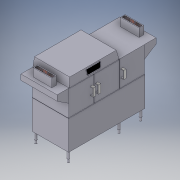
# Autodesk Inventor part: maquinaLAvadoraVajilla480603
Saved by Autodesk Inventor 2018 (Build 220112000, 112)
## iProperties
Created: 2020-04-13
Part Number: maquinaLAvadoraVajilla480603
Material: Generic
Document SubType Name: Modeling
Designer: Jaime
Density: 1 g/cm^3
Appearance: Weld - Stainless Steel
Author: Jaime
Autodesk Inventor part; units mm, degrees
ref_plane "YZ Plane" through (0, 0, 0) normal (1, 0, 0) x (0, 1, 0)
ref_plane "XZ Plane" through (0, 0, 0) normal (0, 1, 0) x (-1, 0, 0)
ref_plane "XY Plane" through (0, 0, 0) normal (0, 0, 1) x (1, 0, 0)
sketch "Sketch1" plane through (0, 0, 0) normal (0, 1, 0) x (-1, 0, 0)
  line L0 (-396.875, 831.85) -> (396.875, 831.85)
  line L1 (396.875, 831.85) -> (396.875, -831.85)
  line L2 (396.875, -831.85) -> (-396.875, -831.85)
  line L3 (-396.875, -831.85) -> (-396.875, 831.85)
  line L4 (-396.875, 831.85) -> (396.875, -831.85) construction
  line L5 (396.875, 831.85) -> (-396.875, -831.85) construction
  point P0 (0, 0)
  dimension "d0" = 793.75
  dimension "d1" = 1663.7
  constraints: 12 end point, 2 midpoint, 2 parallel, 1 horizontal, 1 perpendicular
  measures "d0" distance of L1.end L2.end
  measures "d1" distance of L0.end L1.end
extrude "Extrusion1" add sketch "Sketch1" along normal mid plane 638.175
sketch "Supports" plane through (0, -319.0875, 0) normal (0, -1, 0) x (1, 0, 0)
  line L0 (396.875, 831.85) -> (-396.875, 831.85) construction
  line L1 (-396.875, 831.85) -> (-396.875, -831.85) construction
  line L2 (-396.875, -831.85) -> (396.875, -831.85) construction
  line L3 (396.875, -831.85) -> (396.875, 831.85) construction
  point P0 (0, 0)
sketch "Sketch3" plane through (0, 319.0875, 0) normal (0, 1, 0) x (1, 0, 0)
  line L0 (-396.875, -831.85) -> (396.875, -831.85) construction
  line L1 (396.875, -831.85) -> (396.875, 831.85) construction
  line L2 (396.875, 831.85) -> (-396.875, 831.85) construction
  line L3 (-396.875, 831.85) -> (-396.875, -831.85) construction
  line L4 (-396.875, -825.5) -> (396.875, -825.5)
  line L5 (396.875, -825.5) -> (396.875, 825.5)
  line L6 (396.875, 825.5) -> (-396.875, 825.5)
  line L7 (-396.875, 825.5) -> (-396.875, -825.5)
  line L8 (-396.875, -825.5) -> (396.875, 825.5) construction
  line L9 (396.875, -825.5) -> (-396.875, 825.5) construction
  point P0 (0, 0)
  dimension "d4" = 793.75
  dimension "d5" = 1651
  constraints: 12 end point, 2 midpoint, 2 parallel, 1 horizontal, 1 perpendicular
  measures "d4" distance of L6.end L5.end
  measures "d5" distance of L5.end L4.end
extrude "Extrusion2" add sketch "Sketch3" along normal blind 571.5
sketch "Sketch4" plane through (396.875, -319.0875, -831.85) normal (1, 0, 0) x (0, 0, -1)
  line L0 (0, 638.175) -> (0, 0) construction
  line L1 (-6.35, 638.175) -> (0, 638.175) construction
  line L2 (-6.35, 638.175) -> (-6.35, 1209.675) construction
  line L3 (-1657.35, 1209.675) -> (-6.35, 1209.675) construction
  line L4 (-1657.35, 638.175) -> (-1657.35, 1209.675) construction
  line L5 (-1663.7, 638.175) -> (-1657.35, 638.175) construction
  line L6 (-1663.7, 0) -> (-1663.7, 638.175) construction
  line L7 (0, 0) -> (-1663.7, 0) construction
  line L8 (-1657.35, 638.175) -> (-1657.35, 1209.675) construction
  line L9 (-1657.35, 1209.675) -> (-6.35, 1209.675) construction
  line L10 (-6.35, 1209.675) -> (-6.35, 638.175) construction
  line L11 (-1657.35, 638.175) -> (-1657.35, 1209.675) construction
  line L12 (-1657.35, 1209.675) -> (-6.35, 1209.675) construction
  line L13 (-1657.35, 1209.675) -> (-1107.0167, 1209.675) construction
  line L14 (-1657.35, 1209.675) -> (-1107.0167, 1209.675) construction
  line L15 (-1107.0167, 1209.675) -> (-556.6833, 1209.675) construction
  line L16 (-1107.0167, 1209.675) -> (-556.6833, 1209.675) construction
  line L17 (-556.6833, 1209.675) -> (-6.35, 1209.675) construction
  line L18 (-1107.0167, 1209.675) -> (-1107.0167, 638.175) construction
  line L19 (-556.6833, 1209.675) -> (-556.6833, 638.175) construction
  line L20 (-1113.3667, 638.175) -> (-1100.6667, 638.175)
  line L21 (-1100.6667, 650.875) -> (-1100.6667, 1209.675)
  line L22 (-1100.6667, 1209.675) -> (-1113.3667, 1209.675)
  line L23 (-1113.3667, 1209.675) -> (-1113.3667, 650.875)
  line L24 (-1113.3667, 638.175) -> (-1100.6667, 1209.675) construction
  line L25 (-1100.6667, 638.175) -> (-1113.3667, 1209.675) construction
  line L26 (-563.0333, 638.175) -> (-550.3333, 638.175)
  line L27 (-550.3333, 650.875) -> (-550.3333, 1209.675)
  line L28 (-550.3333, 1209.675) -> (-563.0333, 1209.675)
  line L29 (-563.0333, 1209.675) -> (-563.0333, 650.875)
  line L30 (-563.0333, 638.175) -> (-550.3333, 1209.675) construction
  line L31 (-550.3333, 638.175) -> (-563.0333, 1209.675) construction
  line L32 (-6.35, 638.175) -> (-6.35, 650.875) construction
  line L33 (-6.35, 638.175) -> (6.35, 638.175) construction
  line L34 (-1657.35, 638.175) -> (-6.35, 638.175)
  line L35 (-6.35, 638.175) -> (-6.35, 650.875)
  line L36 (-1657.35, 650.875) -> (-1657.35, 638.175)
  line L37 (-1113.0844, 650.875) -> (-1657.35, 650.875)
  line L38 (-6.35, 638.175) -> (-1107.0167, 638.175) construction
  line L39 (-1113.3667, 638.175) -> (-1657.35, 638.175) construction
  line L40 (-6.35, 650.875) -> (-550.6156, 650.875)
  line L41 (-562.7511, 650.875) -> (-1100.9489, 650.875)
  point P0 (-831.85, 319.0875)
  point P1 (-1107.0167, 923.925)
  point P2 (-556.6833, 923.925)
  dimension "d8" = 550.3333
  dimension "d9" = 0
  dimension "d10" = 550.3333
  dimension "d11" = 0
  dimension "d12" = 12.7
  dimension "d13" = 12.7
  dimension "d16" = 12.7
  dimension "d17" = 90
  dimension "d18" = 1.273
  dimension "d19" = 638.175
  dimension "d20" = 650.875
  dimension "d21" = 638.175
  dimension "d22" = 650.875
  constraints: 64 end point, 12 parallel, 10 point on line, 8 horizontal, 8 perpendicular, 7 midpoint, 3 equal length, 2 collinear, 1 vertical
  measures "d8" distance of L3.start L13.end
  measures "d9" distance between parallel lines of L13 L14
  measures "d10" distance of L14.end L15.end
  measures "d11" distance between parallel lines of L15 L16
  measures "d12" distance of L22.end L21.end
  measures "d13" distance of L28.end L27.end
  measures "d16" distance of L1.start L32.end
  measures "d17" angle of L33 L32
  measures "d18" angle of L0 L30
  measures "d19" distance between parallel lines of L7 L26
  measures "d20" distance between parallel lines of L7 L41
  measures "d21" distance between parallel lines of L7 L34
  measures "d22" distance between parallel lines of L7 L37
extrude "Extrusion3" cut sketch "Sketch4" against normal blind 12.7
sketch "Sketch5" plane through (-396.875, -319.0875, 831.85) normal (-1, 0, 0) x (0, 0, 1)
  line L0 (0, 638.175) -> (0, 0) construction
  line L1 (-6.35, 638.175) -> (0, 638.175) construction
  line L2 (-6.35, 638.175) -> (-6.35, 1209.675) construction
  line L3 (-1657.35, 1209.675) -> (-6.35, 1209.675) construction
  line L4 (-1657.35, 638.175) -> (-1657.35, 1209.675) construction
  line L5 (-1663.7, 638.175) -> (-1657.35, 638.175) construction
  line L6 (-1663.7, 638.175) -> (-1663.7, 0) construction
  line L7 (0, 0) -> (-1663.7, 0) construction
  line L8 (-1657.35, 638.175) -> (-6.35, 638.175) construction
  line L9 (-1657.35, 638.175) -> (-1657.35, 1209.675) projected
  line L10 (-1657.35, 1209.675) -> (-1657.35, 923.925)
  line L11 (-1657.35, 1209.675) -> (-1371.6, 1209.675) construction
  line L12 (-1657.35, 1209.675) -> (-1911.35, 1209.675)
  line L13 (-1657.35, 1209.675) -> (-1403.35, 1209.675) construction
  line L14 (-1911.35, 1209.675) -> (-1911.35, 1089.025)
  line L15 (-1911.35, 1089.025) -> (-1657.35, 923.925)
  line L16 (-1657.35, 1209.675) -> (-6.35, 1209.675) construction
  line L17 (-1657.35, 1209.675) -> (-831.85, 1209.675) construction
  line L18 (-1657.35, 1209.675) -> (-831.85, 1209.675) construction
  line L19 (-831.85, 1209.675) -> (-831.85, 638.175) construction
  line L20 (-6.35, 1209.675) -> (-6.35, 923.925)
  line L21 (-6.35, 1209.675) -> (247.65, 1209.675)
  line L22 (247.65, 1209.675) -> (247.65, 1089.025)
  line L23 (247.65, 1089.025) -> (-6.35, 923.925)
  point P0 (-831.85, 319.0875)
  dimension "d23" = 285.75
  dimension "d24" = 90
  dimension "d25" = 254
  dimension "d26" = 180
  dimension "d27" = 120.65
  dimension "d28" = 90
  dimension "d30" = 825.5
  dimension "d31" = 0
  constraints: 26 end point, 4 horizontal, 3 equal length, 3 symmetric about line, 2 perpendicular, 1 collinear, 1 midpoint
  measures "d23" distance of L3.start L10.end
  measures "d24" angle of L10 L11
  measures "d25" distance of L3.start L12.end
  measures "d26" angle of L12 L13
  measures "d27" distance of L12.end L14.end
  measures "d28" angle of L14 L12
  measures "d30" distance of L3.start L17.end
  measures "d31" distance between parallel lines of L17 L18
extrude "Extrusion4" add sketch "Sketch5" against normal blind 790.575
sketch "Sketch7" plane through (0, 890.5875, 0) normal (0, 1, 0) x (1, 0, 0)
  line L0 (396.875, 268.8167) -> (384.175, 268.8167) construction
  line L1 (384.175, 268.8167) -> (384.175, 281.5167) construction
  line L2 (384.175, 281.5167) -> (396.875, 281.5167) construction
  line L3 (396.875, 281.5167) -> (396.875, 825.5) construction
  line L4 (396.875, 825.5) -> (393.7, 825.5) construction
  line L5 (393.7, 1079.5) -> (393.7, 825.5) construction
  line L6 (-396.875, 1079.5) -> (393.7, 1079.5) construction
  line L7 (-396.875, 1079.5) -> (-396.875, -1079.5) construction
  line L8 (-396.875, -1079.5) -> (393.7, -1079.5) construction
  line L9 (393.7, -825.5) -> (393.7, -1079.5) construction
  line L10 (393.7, -825.5) -> (396.875, -825.5) construction
  line L11 (396.875, -825.5) -> (396.875, -281.5167) construction
  line L12 (396.875, -281.5167) -> (384.175, -281.5167) construction
  line L13 (384.175, -281.5167) -> (384.175, -268.8167) construction
  line L14 (384.175, -268.8167) -> (396.875, -268.8167) construction
  line L15 (396.875, -268.8167) -> (396.875, 268.8167) construction
  line L16 (-396.875, 825.5) -> (393.7, 825.5) construction
  line L17 (393.7, -825.5) -> (-396.875, -825.5) construction
  line L18 (-396.875, 1079.5) -> (393.7, 1079.5) construction
  line L19 (-1.5875, 1079.5) -> (-1.5875, 825.5) construction
  line L20 (-396.875, 825.5) -> (384.175, 825.5) construction
  line L21 (393.7, -825.5) -> (396.875, -825.5) construction
  line L22 (-396.875, -825.5) -> (393.7, -825.5) construction
  line L23 (393.7, 825.5) -> (-396.875, 825.5) construction
  line L24 (-396.875, -831.85) -> (-396.875, 831.85) projected
  line L25 (-396.875, -825.5) -> (-396.875, -831.85) projected
  line L26 (-396.875, -825.5) -> (393.7, -1079.5) construction
  line L27 (393.7, -825.5) -> (-396.875, -1079.5) construction
  line L28 (0, 0) -> (762, 0) construction
  line L29 (0, 0) -> (762, 0) construction
  line L30 (-396.875, -1079.5) -> (-396.875, 1079.5) construction
  line L31 (-396.875, 1079.5) -> (393.7, 1079.5) construction
  line L32 (393.7, 825.5) -> (393.7, 1079.5) construction
  line L33 (393.7, 825.5) -> (396.875, 825.5) construction
  line L34 (396.875, 825.5) -> (396.875, 281.5167) construction
  line L35 (393.7, 825.5) -> (-396.875, 825.5) construction
  line L36 (393.7, 825.5) -> (396.875, 825.5) construction
  line L37 (-396.875, 825.5) -> (393.7, 825.5) construction
  line L38 (-396.875, 831.85) -> (-396.875, -831.85)
  line L39 (-396.875, 825.5) -> (-396.875, 831.85)
  line L40 (-396.875, 825.5) -> (393.7, 1079.5) construction
  line L41 (393.7, 825.5) -> (-396.875, 1079.5) construction
  line L42 (-204.7875, 901.7) -> (201.6125, 901.7)
  line L43 (201.6125, 901.7) -> (201.6125, 1003.3)
  line L44 (201.6125, 1003.3) -> (-204.7875, 1003.3)
  line L45 (-204.7875, 1003.3) -> (-204.7875, 901.7)
  line L46 (-204.7875, 901.7) -> (201.6125, 1003.3) construction
  line L47 (201.6125, 901.7) -> (-204.7875, 1003.3) construction
  line L48 (-204.7875, -1003.3) -> (201.6125, -1003.3)
  line L49 (201.6125, -1003.3) -> (201.6125, -901.7)
  line L50 (201.6125, -901.7) -> (-204.7875, -901.7)
  line L51 (-204.7875, -901.7) -> (-204.7875, -1003.3)
  line L52 (-204.7875, -1003.3) -> (201.6125, -901.7) construction
  line L53 (201.6125, -1003.3) -> (-204.7875, -901.7) construction
  point P0 (-1.5875, 952.5)
  point P1 (-1.5875, -952.5)
  dimension "d34" = 762
  dimension "d35" = 0
  dimension "d36" = 406.4
  dimension "d37" = 101.6
  dimension "d38" = 406.4
  dimension "d39" = 101.6
  constraints: 62 end point, 7 midpoint, 5 perpendicular, 4 horizontal, 4 parallel, 4 symmetric about line, 1 collinear, 1 point on line
  measures "d34" distance of L28.start L28.end
  measures "d35" distance between parallel lines of L28 L29
  measures "d36" distance of L44.end L43.end
  measures "d37" distance of L43.end L42.end
  measures "d38" distance of L50.end L49.end
  measures "d39" distance of L49.end L48.end
extrude "Extrusion5" add sketch "Sketch7" along normal blind 177.8
sketch "Sketch8" plane through (396.875, 331.7875, -268.8167) normal (1, 0, 0) x (0, 0, -1)
  line L0 (-550.3333, 0) -> (-550.3333, 558.8) construction
  line L1 (-1094.3167, 558.8) -> (-550.3333, 558.8) construction
  line L2 (-1094.3167, 0) -> (-1094.3167, 558.8) construction
  line L3 (-1094.3167, 0) -> (-550.3333, 0) construction
  line L4 (0, 0) -> (0, 558.8) construction
  line L5 (-537.6333, 558.8) -> (0, 558.8) construction
  line L6 (-537.6333, 558.8) -> (-537.6333, 0) construction
  line L7 (-537.6333, 0) -> (0, 0) construction
  line L8 (556.6833, -12.7) -> (-1094.3167, -12.7) construction
  line L9 (556.6833, 0) -> (556.6833, -12.7) projected
  line L10 (12.7, 0) -> (556.6833, 0) construction
  line L11 (12.7, 558.8) -> (12.7, 0) construction
  line L12 (0, 558.8) -> (12.7, 558.8) construction
  line L13 (0, 0) -> (0, 558.8) construction
  line L14 (-537.6333, 0) -> (0, 0) construction
  line L15 (-537.6333, 558.8) -> (-537.6333, 0) construction
  line L16 (-550.3333, 558.8) -> (-537.6333, 558.8) construction
  line L17 (-550.3333, 0) -> (-550.3333, 558.8) construction
  line L18 (-1094.3167, 0) -> (-550.3333, 0) construction
  line L19 (-1094.3167, -12.7) -> (-1094.3167, 0) construction
  line L20 (-543.9833, 558.8) -> (-543.9833, 736.6) construction
  line L21 (-543.9833, 558.8) -> (-366.1833, 558.8) construction
  line L22 (-543.9833, 736.6) -> (-35.9833, 736.6)
  line L23 (-543.9833, 736.6) -> (-35.9833, 736.6) construction
  line L24 (0, 0) -> (0, 558.8) construction
  line L25 (-35.9833, 736.6) -> (0, 558.8)
  line L26 (0, 558.8) -> (-543.9833, 558.8)
  line L27 (-550.3333, 558.8) -> (-537.6333, 558.8) projected
  line L28 (-543.9833, 736.6) -> (-543.9833, 558.8) construction
  line L29 (-537.6333, 0) -> (-537.6333, 558.8) construction
  line L30 (6.35, 558.8) -> (-537.6333, 558.8) construction
  line L31 (-1087.9667, 0) -> (-1087.9667, 558.8) construction
  line L32 (-550.3333, 558.8) -> (-1087.9667, 558.8) construction
  line L33 (-550.3333, 558.8) -> (-550.3333, 0) construction
  line L34 (-1100.6667, 558.8) -> (-1100.6667, 0) construction
  line L35 (-1087.9667, 558.8) -> (-1100.6667, 558.8) construction
  line L36 (-1087.9667, 0) -> (-1087.9667, 558.8) construction
  line L37 (-550.3333, 558.8) -> (-550.3333, 0) construction
  line L38 (-537.6333, 558.8) -> (-550.3333, 558.8) construction
  line L39 (-537.6333, 0) -> (-537.6333, 558.8) construction
  line L40 (-543.9833, 558.8) -> (-721.7833, 558.8) construction
  line L41 (-543.9833, 736.6) -> (-1051.9833, 736.6)
  line L42 (-543.9833, 736.6) -> (-1051.9833, 736.6) construction
  line L43 (-1087.9667, 0) -> (-1087.9667, 558.8)
  line L44 (-1051.9833, 736.6) -> (-1087.9667, 558.8)
  line L45 (-1087.9667, 558.8) -> (-543.9833, 558.8)
  line L46 (-537.6333, 558.8) -> (-550.3333, 558.8)
  point P0 (-268.8167, -331.7875)
  dimension "d42" = 177.8
  dimension "d43" = 90
  dimension "d44" = 508
  dimension "d45" = 0
  constraints: 50 end point, 18 symmetric about line, 3 horizontal, 2 collinear, 2 equal length, 1 midpoint, 1 vertical
  measures "d42" distance of L20.start L20.end
  measures "d43" angle of L21 L20
  measures "d44" distance of L20.end L22.end
  measures "d45" distance between parallel lines of L22 L23
extrude "Extrusion6" add sketch "Sketch8" against normal blind 793.75
sketch "Sketch9" plane through (396.875, 331.7875, 825.5) normal (1, 0, 0) x (0, 0, -1)
  line L0 (1094.3167, 0) -> (1094.3167, 558.8) construction
  line L1 (1094.3167, 558.8) -> (1058.3333, 736.6) construction
  line L2 (1058.3333, 736.6) -> (42.3333, 736.6) construction
  line L3 (42.3333, 736.6) -> (6.35, 558.8) construction
  line L4 (0, 558.8) -> (6.35, 558.8) construction
  line L5 (0, 0) -> (0, 558.8) construction
  line L6 (0, 0) -> (543.9833, 0) construction
  line L7 (543.9833, 0) -> (543.9833, 558.8) construction
  line L8 (543.9833, 558.8) -> (556.6833, 558.8) construction
  line L9 (556.6833, 558.8) -> (556.6833, 0) construction
  line L10 (556.6833, 0) -> (1094.3167, 0) construction
  line L11 (0, 558.8) -> (1104.9, 558.8)
  line L12 (1104.9, 558.8) -> (1104.9, 546.1)
  line L13 (1104.9, 546.1) -> (0, 546.1)
  line L14 (0, 546.1) -> (0, 558.8)
  point P0 (825.5, -331.7875)
  dimension "d48" = 1104.9
  dimension "d49" = 12.7
  constraints: 8 end point, 2 parallel, 1 horizontal, 1 perpendicular
  measures "d48" distance of L12.end L13.end
  measures "d49" distance of L11.end L12.end
extrude "Extrusion7" cut sketch "Sketch9" against normal blind 12.7
sketch "Sketch10" plane through (396.875, 1068.3875, 783.1667) normal (1, 0, 0) x (0, 0, -1)
  line L0 (-35.9833, -177.8) -> (1051.9833, -177.8) construction
  line L1 (1051.9833, -177.8) -> (1016, 0) construction
  line L2 (1016, 0) -> (0, 0) construction
  line L3 (0, 0) -> (-35.9833, -177.8) construction
  line L4 (1016, 0) -> (0, 0) projected
  line L5 (0, 0) -> (1051.9833, -177.8) construction
  line L6 (-35.9833, -177.8) -> (-296.3333, -177.8) projected
  line L7 (-35.9833, -177.8) -> (1016, 0) construction
  line L8 (384.1714, -136.6592) -> (631.8286, -136.6592)
  line L9 (660.4, -136.6592) -> (660.4, -35.0592) construction
  line L10 (645.2647, -35.0592) -> (370.7353, -35.0592)
  line L11 (355.6, -35.0592) -> (355.6, -136.6592) construction
  line L12 (355.6, -136.6592) -> (660.4, -35.0592) construction
  line L13 (660.4, -136.6592) -> (355.6, -35.0592) construction
  line L14 (358.2282, -49.9645) -> (371.6643, -126.1645)
  line L15 (355.6, -35.0592) -> (482.6, -35.0592) construction
  line L16 (508, -85.8592) -> (508, -35.0592) construction
  line L17 (657.7718, -49.9645) -> (644.3357, -126.1645)
  arc A0 (370.7353, -35.0592) -> (358.2282, -49.9645) centre (370.7353, -47.7592) ccw
  arc A1 (657.7718, -49.9645) -> (645.2647, -35.0592) centre (645.2647, -47.7592) ccw
  arc A2 (371.6643, -126.1645) -> (384.1714, -136.6592) centre (384.1714, -123.9592) ccw
  arc A3 (631.8286, -136.6592) -> (644.3357, -126.1645) centre (631.8286, -123.9592) ccw
  line L18 (370.7353, -22.3592) -> (645.2647, -22.3592)
  arc A4 (670.2788, -52.1698) -> (645.2647, -22.3592) centre (645.2647, -47.7592) ccw
  line L19 (670.2788, -52.1698) -> (656.8427, -128.3698)
  arc A5 (631.8286, -149.3592) -> (656.8427, -128.3698) centre (631.8286, -123.9592) ccw
  line L20 (631.8286, -149.3592) -> (384.1714, -149.3592)
  arc A6 (359.1573, -128.3698) -> (384.1714, -149.3592) centre (384.1714, -123.9592) ccw
  line L21 (359.1573, -128.3698) -> (345.7212, -52.1698)
  arc A7 (370.7353, -22.3592) -> (345.7212, -52.1698) centre (370.7353, -47.7592) ccw
  point P0 (783.1667, -1068.3875)
  point P1 (373.5148, -136.6592)
  point P2 (642.4852, -136.6592)
  dimension "d56" = 304.8
  dimension "d57" = 101.6
  dimension "d59" = 80
  dimension "d60" = 12.7
  dimension "d61" = 12.7
  dimension "d62" = 12.7
  constraints: 32 end point, 16 point on circle, 11 point on line, 8 centre point, 8 tangent, 3 midpoint, 3 parallel, 2 equal radius, 2 horizontal, 1 perpendicular, 1 symmetric about line, 7 other
  measures "d56" distance of L11.start L9.end
  measures "d57" distance of L9.end L9.start
  measures "d59" angle of L14 L15
  measures "d60" radius of A0
  measures "d61" radius of A1
  measures "d62" distance between parallel lines of L10 L18
ref_plane "Work Plane1" through (371.475, 1068.3875, 783.1667) normal (1, 0, 0) x (0, 0, -1)
sketch "Sketch11" plane through (-396.875, 319.0875, 825.5) normal (0, 0, 1) x (1, 0, 0)
  line L0 (793.75, 749.3) -> (793.75, 571.5) construction
  line L1 (793.75, 749.3) -> (0, 749.3) construction
  line L2 (0, 571.5) -> (0, 749.3) construction
  line L3 (781.05, 571.5) -> (0, 571.5) construction
  line L4 (793.75, 571.5) -> (781.05, 571.5) construction
  line L5 (793.75, 571.5) -> (781.05, 571.5) projected
  line L6 (793.75, 571.5) -> (768.2033, 749.3)
  line L7 (793.75, 749.3) -> (0, 749.3) projected
  line L8 (793.75, 749.3) -> (768.2033, 749.3)
  line L9 (793.75, 571.5) -> (793.75, 749.3) projected
  line L10 (793.75, 749.3) -> (793.75, 571.5)
  point P0 (396.875, -319.0875)
  dimension "d53" = 98.176
  constraints: 6 end point, 1 collinear, 1 point on line, 1 vertical
  measures "d53" angle of L7 L6
extrude "Extrusion8" cut sketch "Sketch11" against normal blind 1092.2
extrude "Extrusion9" cut sketch "Sketch10" against normal blind 76.2
sketch "Sketch12" plane through (0, 1068.3875, 0) normal (0, 1, 0) x (1, 0, 0)
  line L0 (-204.7875, 901.7) -> (201.6125, 901.7) construction
  line L1 (-204.7875, 901.7) -> (201.6125, 901.7) construction
  line L2 (201.6125, 901.7) -> (201.6125, 1003.3) construction
  line L3 (201.6125, 1003.3) -> (-204.7875, 1003.3) construction
  line L4 (-204.7875, 1003.3) -> (-204.7875, 901.7) construction
  line L5 (-204.7875, -1003.3) -> (201.6125, -1003.3) construction
  line L6 (201.6125, -1003.3) -> (201.6125, -901.7) construction
  line L7 (201.6125, -901.7) -> (-204.7875, -901.7) construction
  line L8 (-204.7875, -901.7) -> (-204.7875, -1003.3) construction
  line L9 (-204.7875, -1003.3) -> (201.6125, -901.7) construction
  line L10 (-204.7875, -1003.3) -> (201.6125, -1003.3) construction
  line L11 (201.6125, -1003.3) -> (-204.7875, -901.7) construction
  line L12 (188.9125, -985.52) -> (-192.0875, -985.52)
  line L13 (-192.0875, -985.52) -> (-192.0875, -919.48)
  line L14 (-192.0875, -919.48) -> (188.9125, -919.48)
  line L15 (188.9125, -919.48) -> (188.9125, -985.52)
  line L16 (188.9125, -985.52) -> (-192.0875, -919.48) construction
  line L17 (-192.0875, -985.52) -> (188.9125, -919.48) construction
  line L18 (-204.7875, 901.7) -> (-204.7875, 1003.3) construction
  line L19 (201.6125, 1003.3) -> (-204.7875, 901.7) construction
  line L20 (201.6125, 1003.3) -> (-204.7875, 1003.3) construction
  line L21 (-204.7875, 1003.3) -> (201.6125, 901.7) construction
  line L22 (188.9125, 919.48) -> (-192.0875, 919.48)
  line L23 (-192.0875, 919.48) -> (-192.0875, 985.52)
  line L24 (-192.0875, 985.52) -> (188.9125, 985.52)
  line L25 (188.9125, 985.52) -> (188.9125, 919.48)
  line L26 (188.9125, 919.48) -> (-192.0875, 985.52) construction
  line L27 (-192.0875, 919.48) -> (188.9125, 985.52) construction
  point P0 (0, 0)
  point P1 (-1.5875, -952.5)
  point P2 (-1.5875, 952.5)
  dimension "d65" = 381
  dimension "d66" = 66.04
  dimension "d67" = 381
  dimension "d68" = 66.04
  constraints: 32 end point, 6 midpoint, 4 parallel, 2 horizontal, 2 perpendicular
  measures "d65" distance of L13.end L14.end
  measures "d66" distance of L12.end L13.end
  measures "d67" distance of L23.end L24.end
  measures "d68" distance of L22.end L23.end
extrude "Extrusion10" cut sketch "Sketch12" against normal blind 76.2
sketch "Sketch13" plane through (0, -319.0875, 0) normal (0, -1, 0) x (1, 0, 0)
  line L0 (396.875, 831.85) -> (-396.875, 831.85) construction
  line L1 (-396.875, 831.85) -> (-396.875, -831.85) construction
  line L2 (-396.875, -831.85) -> (396.875, -831.85) construction
  line L3 (396.875, -831.85) -> (396.875, 831.85) construction
  line L4 (396.875, 281.5167) -> (396.875, 825.5) construction
  line L5 (396.875, 825.5) -> (396.875, 281.5167) construction
  line L6 (396.875, -268.8167) -> (396.875, 268.8167) construction
  line L7 (396.875, 268.8167) -> (396.875, -268.8167) construction
  line L8 (396.875, 825.5) -> (396.875, 281.5167) construction
  line L9 (396.875, 825.5) -> (396.875, 281.5167) construction
  line L10 (384.175, 825.5) -> (396.875, 825.5) construction
  line L11 (384.175, 825.5) -> (384.175, 281.5167) construction
  line L12 (396.875, 281.5167) -> (384.175, 281.5167) construction
  line L13 (396.875, 268.8167) -> (396.875, -268.8167) construction
  line L14 (396.875, 268.8167) -> (384.175, 268.8167) construction
  line L15 (384.175, 268.8167) -> (384.175, -268.8167) construction
  line L16 (396.875, -268.8167) -> (384.175, -268.8167) construction
  line L17 (-396.875, -268.8167) -> (384.175, -268.8167) construction
  line L18 (396.875, -268.8167) -> (-396.875, -268.8167) construction
  line L19 (384.175, -268.8167) -> (384.175, 268.8167) construction
  line L20 (384.175, -268.8167) -> (-396.875, -831.85) construction
  line L21 (-396.875, -1079.5) -> (-396.875, -268.8167) construction
  line L22 (396.875, -831.85) -> (396.875, 831.85) construction
  line L23 (-396.875, -268.8167) -> (396.875, -831.85) construction
  line L24 (-358.8006, -313.113) -> (352.3994, -313.113) construction
  line L25 (352.3994, -313.113) -> (352.3994, -783.013) construction
  line L26 (352.3994, -783.013) -> (-358.8006, -783.013) construction
  line L27 (-358.8006, -783.013) -> (-358.8006, -313.113) construction
  line L28 (-358.8006, -313.113) -> (352.3994, -783.013) construction
  line L29 (352.3994, -313.113) -> (-358.8006, -783.013) construction
  circle A0 centre (352.3994, -313.113) radius 25.4
  circle A1 centre (352.3994, -783.013) radius 25.4
  circle A2 centre (-358.8006, -313.113) radius 25.4
  circle A3 centre (-358.8006, -783.013) radius 25.4
  line L30 (352.3994, -783.013) -> (352.3994, 791.787) construction
  line L31 (352.3994, -783.013) -> (1927.1994, -783.013) construction
  line L32 (-358.8006, -783.013) -> (-358.8006, 791.787) construction
  line L33 (-358.8006, -783.013) -> (1215.9994, -783.013) construction
  circle A4 centre (352.3994, 791.787) radius 25.4
  circle A5 centre (-358.8006, 791.787) radius 25.4
  point P0 (0, 0)
  point P1 (-3.2006, -548.063)
  dimension "d71" = 711.2
  dimension "d72" = 469.9
  dimension "d73" = 50.8
  dimension "d74" = 50.8
  dimension "d75" = 50.8
  dimension "d76" = 50.8
  dimension "d77" = 1574.8
  dimension "d78" = 90
  dimension "d79" = 1574.8
  dimension "d80" = 90
  dimension "d81" = 50.8
  dimension "d82" = 50.8
  constraints: 26 end point, 6 centre point, 6 coincident, 3 horizontal, 3 perpendicular, 2 midpoint, 2 parallel, 2 point on line, 2 vertical, 1 collinear, 1 other
  measures "d71" distance of L25.end L26.end
  measures "d72" distance of L24.end L25.end
  measures "d73" diameter of A0
  measures "d74" diameter of A1
  measures "d75" diameter of A2
  measures "d76" diameter of A3
  measures "d77" distance of L30.start L30.end
  measures "d78" angle of L31 L30
  measures "d79" distance of L32.start L32.end
  measures "d80" angle of L33 L32
  measures "d81" diameter of A4
  measures "d82" diameter of A5
extrude "Extrusion11" add sketch "Sketch13" along normal blind 152.4
sketch "Sketch14" plane through (352.3994, -471.4875, -313.113) normal (0, -1, 0) x (1, 0, 0)
  line L0 (18.9289, 1096.2797) -> (-749.2744, 1096.2797) construction
  circle A0 centre (0, 1104.9) radius 25.4 construction
  circle A1 centre (0, 1104.9) radius 25.4 construction
  circle A2 centre (-711.2, 0) radius 25.4 construction
  circle A3 centre (0, 0) radius 25.4 construction
  circle A4 centre (0, -469.9) radius 25.4 construction
  circle A5 centre (-711.2, -469.9) radius 25.4 construction
  circle A6 centre (-711.2, 1104.9) radius 25.4 construction
  line L1 (44.4756, 1144.963) -> (-749.2744, 1144.963) construction
  line L2 (-749.2744, 1144.963) -> (-749.2744, -518.737) construction
  line L3 (-749.2744, -518.737) -> (44.4756, -518.737) construction
  line L4 (44.4756, -518.737) -> (44.4756, 1144.963) construction
  circle A7 centre (0, -469.9) radius 20.32
  circle A8 centre (0, 0) radius 20.32
  circle A9 centre (-711.2, -469.9) radius 20.32
  circle A10 centre (-711.2, 0) radius 20.32
  circle A11 centre (-711.2, 1104.9) radius 20.32
  circle A12 centre (0, 1104.9) radius 20.32
  point P0 (-352.3994, 313.113)
  dimension "d85" = 40.64
  dimension "d86" = 40.64
  dimension "d87" = 40.64
  dimension "d88" = 40.64
  dimension "d89" = 40.64
  dimension "d90" = 40.64
  constraints: 6 centre point, 6 coincident
  measures "d85" diameter of A7
  measures "d86" diameter of A8
  measures "d87" diameter of A9
  measures "d88" diameter of A10
  measures "d89" diameter of A11
  measures "d90" diameter of A12
extrude "Extrusion12" add sketch "Sketch14" along normal blind 73.025
sketch "Sketch15" plane through (396.875, 331.7875, 825.5) normal (1, 0, 0) x (0, 0, -1)
  line L0 (543.9833, 546.1) -> (0, 546.1) construction
  line L1 (0, 0) -> (0, 546.1) construction
  line L2 (0, 0) -> (543.9833, 0) construction
  line L3 (543.9833, 0) -> (543.9833, 546.1) construction
  line L4 (1094.3167, 546.1) -> (556.6833, 546.1) construction
  line L5 (556.6833, 546.1) -> (556.6833, 0) construction
  line L6 (556.6833, 0) -> (1094.3167, 0) construction
  line L7 (1094.3167, 0) -> (1094.3167, 546.1) construction
  line L8 (1107.0167, 558.8) -> (1107.0167, 0) construction
  line L9 (1107.0167, 0) -> (1651, 0) construction
  line L10 (1651, 0) -> (1651, 558.8) construction
  line L11 (1107.0167, 558.8) -> (1651, 558.8) construction
  line L12 (543.9833, 546.1) -> (543.9833, 273.05) construction
  line L13 (543.9833, 0) -> (543.9833, 546.1) construction
  line L14 (543.9833, 273.05) -> (556.6833, 273.05) construction
  line L15 (556.6833, 546.1) -> (556.6833, 0) construction
  line L16 (1107.0167, 558.8) -> (1107.0167, 0) construction
  line L17 (556.6833, 273.05) -> (1107.0167, 273.05) construction
  line L18 (543.9833, 273.05) -> (493.1833, 273.05) construction
  line L19 (543.9833, 273.05) -> (594.7833, 273.05) construction
  line L20 (556.6833, 273.05) -> (607.4833, 273.05) construction
  line L21 (556.6833, 273.05) -> (607.4833, 273.05) construction
  line L22 (1107.0167, 273.05) -> (1157.8167, 273.05) construction
  line L23 (1094.3167, 0) -> (1094.3167, 546.1) construction
  line L24 (1107.0167, 273.05) -> (1157.8167, 273.05) construction
  line L25 (467.7833, 184.15) -> (518.5833, 184.15)
  line L26 (518.5833, 184.15) -> (518.5833, 361.95)
  line L27 (518.5833, 361.95) -> (467.7833, 361.95)
  line L28 (467.7833, 361.95) -> (467.7833, 184.15)
  line L29 (467.7833, 184.15) -> (518.5833, 361.95) construction
  line L30 (518.5833, 184.15) -> (467.7833, 361.95) construction
  line L31 (582.0833, 184.15) -> (632.8833, 184.15)
  line L32 (632.8833, 184.15) -> (632.8833, 361.95)
  line L33 (632.8833, 361.95) -> (582.0833, 361.95)
  line L34 (582.0833, 361.95) -> (582.0833, 184.15)
  line L35 (582.0833, 184.15) -> (632.8833, 361.95) construction
  line L36 (632.8833, 184.15) -> (582.0833, 361.95) construction
  line L37 (1132.4167, 184.15) -> (1183.2167, 184.15)
  line L38 (1183.2167, 184.15) -> (1183.2167, 361.95)
  line L39 (1183.2167, 361.95) -> (1132.4167, 361.95)
  line L40 (1132.4167, 361.95) -> (1132.4167, 184.15)
  line L41 (1132.4167, 184.15) -> (1183.2167, 361.95) construction
  line L42 (1183.2167, 184.15) -> (1132.4167, 361.95) construction
  point P0 (825.5, -331.7875)
  dimension "d93" = 273.05
  dimension "d94" = 50.8
  dimension "d95" = 180
  dimension "d96" = 50.8
  dimension "d97" = 0
  dimension "d98" = 50.8
  dimension "d99" = 0
  dimension "d100" = 50.8
  dimension "d101" = 177.8
  dimension "d102" = 50.8
  dimension "d103" = 177.8
  dimension "d104" = 50.8
  dimension "d105" = 177.8
  constraints: 54 end point, 8 midpoint, 7 equal length, 6 horizontal, 6 perpendicular, 3 collinear, 1 point on line
  measures "d93" distance of L0.start L12.end
  measures "d94" distance of L12.end L18.end
  measures "d95" angle of L18 L19
  measures "d96" distance of L14.end L20.end
  measures "d97" distance between parallel lines of L20 L21
  measures "d98" distance of L17.end L22.end
  measures "d99" distance between parallel lines of L22 L24
  measures "d100" distance of L27.end L26.end
  measures "d101" distance of L26.end L25.end
  measures "d102" distance of L33.end L32.end
  measures "d103" distance of L32.end L31.end
  measures "d104" distance of L39.end L38.end
  measures "d105" distance of L38.end L37.end
extrude "Extrusion13" add sketch "Sketch15" along normal blind 63.5
sketch "Sketch16" plane through (396.875, 515.9375, -357.7167) normal (0, 0, -1) x (-1, 0, 0)
  line L0 (0, 177.8) -> (0, 0) construction
  line L1 (0, 177.8) -> (-63.5, 177.8) construction
  line L2 (-63.5, 0) -> (-63.5, 177.8) construction
  line L3 (0, 0) -> (-63.5, 0) construction
  line L4 (-63.5, 177.8) -> (0, 0) construction
  line L5 (0, 0) -> (-63.5, 0) construction
  line L6 (-63.5, 0) -> (0, 177.8) construction
  line L7 (-31.75, 88.9) -> (-21.59, 88.9) construction
  line L8 (-31.75, 88.9) -> (-21.59, 88.9) construction
  line L9 (0, 177.8) -> (0, 165.1) construction
  line L10 (0, -184.15) -> (0, 361.95) construction
  line L11 (0, 177.8) -> (12.7, 177.8) construction
  line L12 (0, 165.1) -> (-50.8, 165.1) construction
  line L13 (-50.8, 165.1) -> (0, 0) construction
  line L14 (0, 0) -> (0, 12.7) construction
  line L15 (0, 0) -> (12.7, 0) construction
  line L16 (0, 12.7) -> (-50.8, 12.7)
  line L17 (-50.8, 12.7) -> (-50.8, 165.1)
  line L18 (-50.8, 165.1) -> (0, 165.1)
  line L19 (0, 165.1) -> (0, 12.7)
  point P0 (396.875, -515.9375)
  dimension "d108" = 10.16
  dimension "d109" = 0
  dimension "d110" = 12.7
  dimension "d111" = 90
  dimension "d112" = 50.8
  dimension "d113" = 90
  dimension "d114" = 12.7
  dimension "d115" = 90
  constraints: 28 end point, 5 horizontal, 3 equal length, 2 parallel, 2 perpendicular, 1 collinear, 1 midpoint, 1 vertical
  measures "d108" distance of L7.start L7.end
  measures "d109" distance between parallel lines of L7 L8
  measures "d110" distance of L0.start L9.end
  measures "d111" angle of L9 L11
  measures "d112" distance of L9.end L12.end
  measures "d113" angle of L9 L12
  measures "d114" distance of L0.end L14.end
  measures "d115" angle of L15 L14
extrude "Extrusion14" cut sketch "Sketch16" against normal blind 762
body "Solid1"
